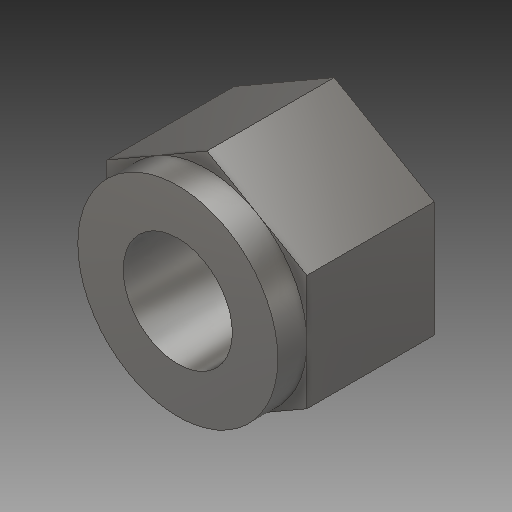
# Autodesk Inventor part: ナイロンナットm3
Saved by Autodesk Inventor 2020 (Build 240168000, 168)
## iProperties
Part Number: ナイロンナットm3
Material: 鉄、可鍛鉄
Document SubType Name: Modeling
Designer: 雪村
Density: 7.15 g/cm^3
Appearance: 半つや出し
Mass: 0.57416 g
Surface Area: 1.59291 cm^2
Volume: 0.0803022 cm^3
Author: 雪村
Autodesk Inventor part; units mm, degrees
ref_plane "YZ Plane" through (0, 0, 0) normal (1, 0, 0) x (0, 1, 0)
ref_plane "XZ Plane" through (0, 0, 0) normal (0, 1, 0) x (-1, 0, 0)
ref_plane "XY Plane" through (0, 0, 0) normal (0, 0, 1) x (1, 0, 0)
sketch "スケッチ1" plane through (0, 0, 0) normal (0, 0, 1) x (1, 0, 0)
  line L0 (0, 3.1754) -> (2.75, 1.5877)
  line L1 (2.75, 1.5877) -> (2.75, -1.5877)
  line L2 (2.75, -1.5877) -> (0, -3.1754)
  line L3 (0, -3.1754) -> (-2.75, -1.5877)
  line L4 (-2.75, -1.5877) -> (-2.75, 1.5877)
  line L5 (-2.75, 1.5877) -> (0, 3.1754)
  point P0 (0, 0)
  point P1 (0, 0)
  dimension "d0" = 5.5
  constraints: 12 end point, 1 coincident, 1 vertical, 13 other
  measures "d0" distance between parallel lines of L1 L4
extrude "押し出し1" add sketch "スケッチ1" along normal blind 3.5
sketch "スケッチ2" plane through (0, 0, 3.5) normal (0, 0, 1) x (1, 0, 0)
  circle A0 centre (0, 0) radius 2.75
  constraints: 1 centre point, 1 coincident
extrude "押し出し2" add sketch "スケッチ2" along normal blind 0.8
sketch "スケッチ3" plane through (0, 0, 4.3) normal (0, 0, 1) x (1, 0, 0)
  circle A0 centre (0, 0) radius 1.5
  dimension "d5" = 3
  constraints: 1 centre point, 1 coincident
  measures "d5" diameter of A0
extrude "押し出し3" cut sketch "スケッチ3" against normal through all
